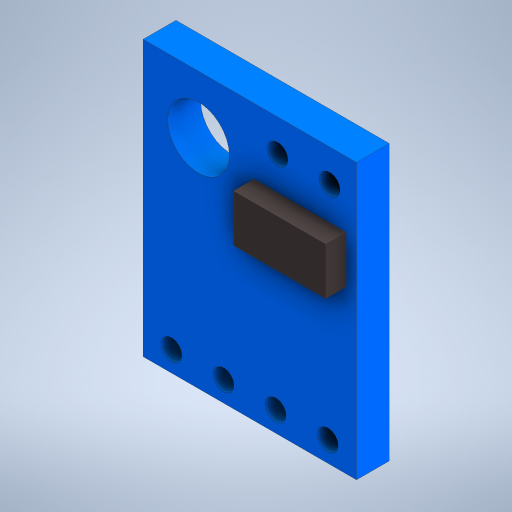
# Autodesk Inventor part: vl53l0x
Saved by Autodesk Inventor 2023 (Build 270158000, 158)
## iProperties
Created: 2024-03-04
Part Number: vl53l0x
Material: Generic
Document SubType Name: Modeling
Designer: pavel
Density: 1 g/cm^3
Appearance: Default
Author: pavel
Autodesk Inventor part; units mm, degrees
ref_plane "YZ Plane" through (0, 0, 0) normal (1, 0, 0) x (0, 1, 0)
ref_plane "XZ Plane" through (0, 0, 0) normal (0, 1, 0) x (-1, 0, 0)
ref_plane "XY Plane" through (0, 0, 0) normal (0, 0, 1) x (1, 0, 0)
sketch "Sketch1" plane through (0, 0, 0) normal (0, 0, 1) x (1, 0, 0)
  line L0 (0, 0) -> (10.4, 0)
  line L1 (10.4, 0) -> (10.4, 13.4)
  line L2 (10.4, 13.4) -> (0, 13.4)
  line L3 (0, 13.4) -> (0, 0)
  dimension "d0" = 10.4
  dimension "d1" = 13.4
  constraints: 8 end point, 2 parallel, 1 horizontal, 1 perpendicular
  measures "d0" distance of L2.end L1.end
  measures "d1" distance of L1.end L0.end
extrude "Extrusion1" add sketch "Sketch1" along normal blind 1.6
sketch "Sketch2" plane through (0, 0, 1.6) normal (0, 0, 1) x (1, 0, 0)
  line L0 (10.4, 13.4) -> (0, 13.4) projected
  line L1 (0, 13.4) -> (0, 0) projected
  point P0 (2.7, 10.6)
  dimension "d4" = 2.8
  dimension "d5" = 2.7
  measures "d4" distance from line of L0 point (2.7, 10.6)
  measures "d5" distance from line of L1 point (2.7, 10.6)
hole "Hole1" at (2.7, 10.6, 1.6) direction (0, 0, -1) diameter 3 depth 1.6
sketch "Sketch3" plane through (0, 0, 1.6) normal (0, 0, 1) x (1, 0, 0)
  line L0 (0, 13.4) -> (0, 0) projected
  line L1 (10.4, 0) -> (10.4, 13.4) projected
  line L2 (0, 0) -> (10.4, 0) projected
  point P0 (1.39, 1)
  point P1 (3.93, 1)
  point P2 (6.47, 1)
  point P3 (9.01, 1)
  point P4 (6.56, 11.8363)
  point P5 (9.1, 11.8363)
  dimension "d13" = 2.54
  dimension "d14" = 2.54
  dimension "d15" = 2.54
  dimension "d16" = 1.39
  dimension "d17" = 2.54
  dimension "d18" = 1.3
  dimension "d19" = 1
  measures "d13" distance of point (3.93, 1) point (1.39, 1)
  measures "d14" distance of point (3.93, 1) point (6.47, 1)
  measures "d15" distance of point (9.01, 1) point (6.47, 1)
  measures "d16" distance from line of L0 point (1.39, 1)
  measures "d17" distance of point (9.1, 11.836) point (6.56, 11.836)
  measures "d18" distance from line of L1 point (9.1, 11.836)
  measures "d19" distance from line of L2 point (1.39, 1)
hole "Hole2" at (1.39, 1, 1.6) at (3.93, 1, 1.6) at (6.47, 1, 1.6) at (9.01, 1, 1.6) at (6.56, 11.8363, 1.6) at (9.1, 11.8363, 1.6) direction (0, 0, -1) diameter 1 end through all
sketch "Sketch4" plane through (0, 0, 1.6) normal (0, 0, 1) x (1, 0, 0)
  line L0 (5.4, 7.9) -> (9.9, 7.9)
  line L1 (9.9, 7.9) -> (9.9, 10.2)
  line L2 (9.9, 10.2) -> (5.4, 10.2)
  line L3 (5.4, 10.2) -> (5.4, 7.9)
  line L4 (10.4, 0) -> (10.4, 13.4) projected
  line L5 (10.4, 13.4) -> (0, 13.4) projected
  point P0 (0, 0)
  dimension "d27" = 4.5
  dimension "d28" = 2.3
  dimension "d29" = 0.5
  dimension "d30" = 3.2
  constraints: 8 end point, 2 parallel, 1 horizontal, 1 perpendicular
  measures "d27" distance of L2.end L1.end
  measures "d28" distance of L1.end L0.end
  measures "d29" distance between parallel lines of L4 L1
  measures "d30" distance between parallel lines of L2 L5
extrude "Extrusion2" add sketch "Sketch4" along normal blind 1
body "Solid1"
